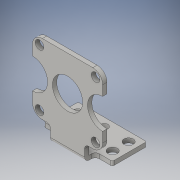
# Autodesk Inventor part: mcdave_mount
Saved by Autodesk Inventor 2016 (Build 200138000, 138)
## iProperties
Created: 2017-09-05
Part Number: mcdave_mount
Material: Generic
Document SubType Name: Modeling
Designer: student
Density: 1 g/cm^3
Appearance: Default
Author: student
Autodesk Inventor part; units mm, degrees
ref_plane "YZ Plane" through (0, 0, 0) normal (1, 0, 0) x (0, 1, 0)
ref_plane "XZ Plane" through (0, 0, 0) normal (0, 1, 0) x (-1, 0, 0)
ref_plane "XY Plane" through (0, 0, 0) normal (0, 0, 1) x (1, 0, 0)
sketch "Sketch1" plane through (0, 0, 0) normal (0, 0, 1) x (1, 0, 0)
  line L0 (-8.8422, 6.5161) -> (13.7638, 6.5161)
  line L1 (13.7638, -16.0899) -> (-8.8422, -16.0899)
  circle A0 centre (2.4608, -4.7869) radius 4.8768
  arc A1 (-8.8422, -9.6637) -> (-8.8422, 0.0899) centre (-8.8422, -4.7869) ccw
  line L2 (-8.8422, -16.0899) -> (-8.8422, -9.6637)
  line L3 (-8.8422, 0.0899) -> (-8.8422, 6.5161)
  arc A2 (13.7638, 0.0899) -> (13.7638, -9.6637) centre (13.7638, -4.7869) ccw
  line L4 (13.7638, 6.5161) -> (13.7638, 0.0899)
  line L5 (13.7638, -9.6637) -> (13.7638, -16.0899)
  dimension "d2" = 22.606
  dimension "d3" = 22.606
  dimension "d4" = 9.7536
  dimension "d5" = 9.7536
  constraints: 12 end point, 5 parallel, 4 point on circle, 3 centre point, 2 perpendicular, 1 horizontal
  measures "d2" distance of L0.end L1.start
  measures "d3" distance of L0.start L0.end
  measures "d4" diameter of A0
  measures "d5" diameter of A1
extrude "Extrusion1" add sketch "Sketch1" along normal blind 1.397
fillet "Fillet1" radius 3.175 4 edges at (-8.8422, 6.5161, 0.6985) (13.7638, 6.5161, 0.6985) (13.7638, -16.0899, 0.6985) (-8.8422, -16.0899, 0.6985)
sketch "Sketch2" plane through (0, 0, 1.397) normal (0, 0, 1) x (1, 0, 0)
  line L0 (-8.8422, 3.3411) -> (-8.8422, 0.0899) projected
  circle A0 centre (-6.5606, 4.3162) radius 1.397
  line L1 (10.5888, 6.5161) -> (-5.6672, 6.5161) projected
  arc A1 (-8.8422, -9.6637) -> (-8.8422, 0.0899) centre (-8.8422, -4.7869) ccw projected
  arc A2 (13.7638, 0.0899) -> (13.7638, -9.6637) centre (13.7638, -4.7869) ccw projected
  circle A3 centre (-6.5606, -13.89) radius 1.397
  line L2 (-5.6672, -16.0899) -> (10.5888, -16.0899) projected
  circle A4 centre (11.4822, 4.3162) radius 1.397
  circle A5 centre (11.4822, -13.89) radius 1.397
  point P0 (0, 0)
  dimension "d9" = 2.794
  constraints: 4 centre point
  measures "d9" diameter of A0
extrude "Extrusion2" cut sketch "Sketch2" against normal blind 1.397
sketch "Sketch3" plane through (0, 0, 1.397) normal (0, 0, 1) x (1, 0, 0)
  line L0 (2.4608, -16.0899) -> (2.4608, -9.6637)
  circle A0 centre (2.4608, -4.7869) radius 4.8768 projected
  line L1 (2.4608, -16.0899) -> (0.1367, -16.0899)
  line L2 (-3.0383, -16.0899) -> (7.9599, -16.0899)
  line L3 (2.4608, -16.0899) -> (7.9599, -16.0899)
  line L4 (2.4608, -16.0899) -> (7.9599, -16.0899)
  line L5 (10.5888, -16.0899) -> (-5.6672, -16.0899) projected
  line L6 (7.9599, -17.9949) -> (7.9599, -16.0899)
  line L7 (-3.0383, -17.9949) -> (-3.0383, -16.0899)
  line L8 (-3.0383, -17.9949) -> (-3.0383, -19.8999)
  line L9 (-3.0383, -19.8999) -> (7.9599, -19.8999)
  line L10 (7.9599, -19.8999) -> (7.9599, -17.9949)
  point P0 (0, 0)
  point P1 (-5.6672, -16.0899)
  dimension "d12" = 5.4991
  dimension "d13" = 5.4991
  dimension "d14" = 1.905
  dimension "d16" = 1.905
  constraints: 20 end point, 3 symmetric about line, 2 perpendicular, 1 collinear, 1 horizontal, 1 point on line, 1 vertical, 1 vertical alignment, 1 other
  measures "d12" distance of L2.start L0.start
  measures "d13" distance of L2.end L0.start
  measures "d14" distance of L2.start L7.start
  measures "d16" distance of L7.start L8.end
extrude "Extrusion3" add sketch "Sketch3" against normal blind 1.397 contours L2 L6 L10 L9 L8 L7 L1
fillet "Fillet2" radius 1.27 2 edges at (7.9599, -16.0899, 0.6985) (-3.0383, -16.0899, 0.6985)
sketch "Sketch4" plane through (-3.0383, -19.8999, 1.397) normal (0, -1, 0) x (1, 0, 0)
  line L0 (10.9982, -1.397) -> (0, -1.397) projected
  line L1 (10.9982, -1.397) -> (10.9982, -3.4544)
  line L2 (10.9982, -3.4544) -> (0, -3.4544)
  line L3 (0, -3.4544) -> (0, -1.397)
  point P0 (3.0383, -1.397)
  dimension "d20" = 2.0574
  constraints: 6 end point, 1 horizontal, 1 perpendicular, 1 vertical
  measures "d20" distance of L0.start L1.end
extrude "Extrusion4" add sketch "Sketch4" along normal blind 1.397
sketch "Sketch5" plane through (-3.0383, -19.8999, 1.397) normal (0, 1, 0) x (1, 0, 0)
  line L0 (10.9982, 3.4544) -> (10.9982, 1.397) projected
  line L1 (10.9982, 3.4544) -> (-5.5499, 3.4544)
  line L2 (-5.5499, 3.4544) -> (-5.5499, 14.4526)
  line L3 (-5.5499, 14.4526) -> (16.4973, 14.4526)
  line L4 (10.9982, 1.397) -> (0, 1.397) projected
  line L5 (0, 3.4544) -> (10.9982, 3.4544) projected
  line L6 (0, 3.4544) -> (10.9982, 3.4544) projected
  line L7 (16.4973, 14.4526) -> (16.4973, 3.4544)
  line L8 (16.4973, 3.4544) -> (10.9982, 3.4544)
  point P0 (5.4991, 3.4544)
  point P1 (5.4991, 3.4544)
  dimension "d25" = 22.0472
  dimension "d38" = 10.9982
  constraints: 10 end point, 2 midpoint, 2 perpendicular, 2 point on line, 1 horizontal, 1 parallel, 1 vertical
  measures "d25" distance of L2.end L3.end
  measures "d38" distance of L1.end L2.end
extrude "Extrusion5" add sketch "Sketch5" against normal blind 1.397
fillet "Fillet3" radius 1.27 2 edges at (-3.0383, -20.5984, -2.0574) (7.9599, -20.5984, -2.0574)
fillet "Fillet4" radius 0.508 4 edges at (-8.5882, -20.5984, -2.0574) (-8.5882, -20.5984, -13.0556) (13.459, -20.5984, -2.0574) (13.459, -20.5984, -13.0556)
sketch "Sketch8" plane through (-3.0383, -19.8999, 0) normal (0, 0, 1) x (1, 0, 0)
  line L0 (0, 0) -> (0, -1.397) projected
  line L1 (0, -1.397) -> (0, 0)
  line L2 (10.9982, 0) -> (10.9982, -1.397) projected
  line L3 (0, 0) -> (10.9982, 0)
  line L4 (10.9982, 0) -> (10.9982, -1.397)
  line L5 (10.9982, -1.397) -> (0, -1.397)
  point P0 (3.0383, 19.8999)
  constraints: 8 end point, 2 perpendicular, 1 collinear, 1 vertical
extrude "Extrusion8" add sketch "Sketch8" along normal blind 1.397
fillet "Fillet5" radius 1.524 1 edges at (2.4608, -21.2969, 1.397)
sketch "Sketch11" plane through (-3.0383, -19.8999, 1.397) normal (0, 1, 0) x (1, 0, 0)
  line L0 (-5.0419, 14.4526) -> (15.9893, 14.4526) projected
  line L1 (-2.6289, 1.397) -> (13.6271, 1.397) projected
  line L2 (16.4973, 13.9446) -> (16.4973, 3.9624) projected
  line L3 (-5.5499, 13.9446) -> (-5.5499, 3.9624) projected
  circle A0 centre (13.6271, 11.5283) radius 1.5113
  line L4 (6.7183, 3.3528) -> (6.7183, 11.811)
  line L5 (4.2291, 11.811) -> (4.2291, 3.3528)
  arc A1 (4.2291, 3.3528) -> (6.7183, 3.3528) centre (5.4737, 3.3528) ccw
  arc A2 (6.7183, 11.811) -> (4.2291, 11.811) centre (5.4737, 11.811) ccw
  circle A3 centre (13.6271, 6.3787) radius 1.5113
  line L6 (0, 1.524) -> (10.9982, 1.524) projected
  circle A4 centre (-2.6681, 11.4963) radius 1.5113
  circle A5 centre (-2.6479, 6.3467) radius 1.5113
  point P0 (5.4737, 7.5819)
  dimension "d43" = 3.0226
  dimension "d47" = 2.8702
  dimension "d50" = 2.6416
  dimension "d51" = 1.9558
  constraints: 6 centre point, 4 end point, 4 point on circle, 4 tangent, 1 parallel
  measures "d43" diameter of A0
  measures "d47" distance from line of L2 A0.centre
  measures "d50" distance from line of L0 A2.centre
  measures "d51" distance from line of L1 A1.centre
extrude "Extrusion10" cut sketch "Sketch11" against normal through all
body "Solid1"
